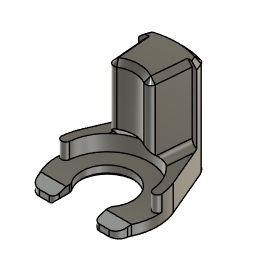
e3d_collet_clip (Autodesk Fusion 360 design; units mm, degrees)
Autodesk Fusion 360 part; units mm, degrees
sketch "Sketch1" plane through (0, 0, 0) normal (0, 0, 1) x (1, 0, 0)
  circle A0 centre (0, 0) radius 2.575
  circle A1 centre (0, 0) radius 5.0605
  line L0 (0, 0) -> (0, 7.5) construction
  line L1 (-2, -1.62192) -> (-2, -3.32192)
  line L2 (-4.4855, -2.342851) -> (-4.4855, -3.32192)
  line L3 (-4.4855, -3.32192) -> (-2, -3.32192)
  line L4 (4.4855, -2.342851) -> (4.4855, -3.32192)
  line L5 (4.4855, -3.32192) -> (2, -3.32192)
  line L6 (2, -1.62192) -> (2, -3.32192)
  arc A2 (2.5, 7.071068) -> (-2.5, 7.071068) centre (0, 0) ccw
  circle A3 centre (0, 0) radius 7.5 construction
  line L7 (-2.5, 7.071068) -> (-4.659517, 1.974223)
  line L8 (2.5, 7.071068) -> (4.659517, 1.974223)
  dimension "d1" = 5.15
  dimension "d2" = 2.4855
  dimension "d13" = 2.4855
  dimension "d18" = 2
  dimension "d20" = 1.7
  dimension "d37" = 15
  dimension "d41" = 5
  constraint coincident A0.centre A1.centre
  constraint concentric A0 A1
  constraint vertical L0
  constraint vertical L1
  constraint vertical L2
  constraint perpendicular L2 L3
  constraint concentric A2 A3
  constraint midpoint L0.end A2
  constraint tangent A1 L7
  constraint tangent A1 L8
  measures "d1" diameter of A0
  measures "d2" distance of A0 A1
  measures "d18" distance of L0 L1
  measures "d37" diameter of A3
extrude "Extrude1" add sketch "Sketch1" along normal blind 1 contours A0 A1 L1 L3 L5 L6 | A1 L2 L3 | A1 L4 L5 | A1 A2 L7 L8 picked at (2.605842, -2.755253) picked at (-4.279884, -3.007191) picked at (4.279884, -3.007191) picked at (0, 6.675289)
sketch "Sketch3" plane through (0, 0, 1) normal (0, 0, 1) x (-1, 0, 0)
  line L0 (2.5, -7.071068) -> (4.659517, -1.974223)
  arc A0 (4.659517, -1.974223) -> (4.4855, 2.342851) centre (0, 0) ccw
  line L1 (4.4855, 2.342851) -> (4.4855, 3.32192)
  line L2 (4.4855, 3.32192) -> (2, 3.32192)
  line L3 (2, 3.32192) -> (2, 1.62192)
  arc A1 (-2, 1.62192) -> (2, 1.62192) centre (0, 0) ccw
  line L4 (-2, 1.62192) -> (-2, 3.32192)
  line L5 (-2, 3.32192) -> (-4.4855, 3.32192)
  line L6 (-4.4855, 3.32192) -> (-4.4855, 2.342851)
  arc A2 (-4.4855, 2.342851) -> (-4.659517, -1.974223) centre (0, 0) ccw
  line L7 (-4.659517, -1.974223) -> (-2.5, -7.071068)
  arc A3 (-2.5, -7.071068) -> (2.5, -7.071068) centre (0, 0) ccw
  arc A4 (-2, 1.62192) -> (2, 1.62192) centre (0, 0) ccw
  arc A5 (-1.367588, -2.328025) -> (1.367588, -2.328025) centre (0, 0) ccw
  arc A6 (-4.185371, -0.3889) -> (4.185371, -0.3889) centre (0, 0) ccw
  arc A7 (5.038794, -0.4682) -> (4.185371, -0.3889) centre (4.612083, -0.42855) ccw
  arc A8 (-4.185371, -0.3889) -> (-5.038794, -0.4682) centre (-4.612083, -0.42855) ccw
  line L8 (5.0605, 0) -> (-5.0605, 0) construction
  line L9 (2.5, -7.071068) -> (2.118943, -2.715563)
  arc A9 (2.118943, -2.715563) -> (1.367588, -2.328025) centre (1.620845, -2.759141) ccw
  arc A10 (-1.367588, -2.328025) -> (-2.118943, -2.715563) centre (-1.620845, -2.759141) ccw
  line L10 (-2.118943, -2.715563) -> (-2.5, -7.071068)
  line L11 (2.5, -7.071068) -> (-2.5, -7.071068) construction
  line L12 (0, 0) -> (0, -7.071068) construction
  line L13 (-2, 1.62192) -> (-2, 3.32192)
  line L14 (2, 3.32192) -> (2, 1.62192)
  line L15 (2, 3.32192) -> (-2, 3.32192)
  line L16 (2.917598, -6.085463) -> (2.417598, -6.129207)
  line L17 (-2.417598, -6.129207) -> (-2.917598, -6.085463)
  dimension "d81" = 2.7
  dimension "d82" = 4.2034
  dimension "d108" = 85
  dimension "d109" = 0.5
  dimension "d125" = 0.5
  dimension "d127" = 0.42855
  constraint coincident A0.centre A1.centre
  constraint tangent A6 A7
  constraint tangent A0 A7
  constraint tangent A6 A8
  constraint tangent A2 A8
  constraint coincident A0 L8.start
  constraint coincident A2 L8.end
  constraint horizontal L8
  constraint coincident A0.centre L8
  constraint tangent A7 L8
  constraint tangent A8 L8
  constraint tangent L9 A9
  constraint tangent A5 A10
  constraint tangent A5 A9
  constraint tangent A10 L10
  constraint symmetric L9 L10 L12
  constraint symmetric A9 A10 L12
  constraint perpendicular L9 L16
  constraint perpendicular L10 L17
  constraint symmetric L12 L16 L17
  measures "d81" radius of A5
  measures "d82" radius of A6
  measures "d108" angle of L9 L11
  measures "d109" radius of A9
  measures "d127" radius of A7
extrude "Extrude5" add sketch "Sketch3" along normal blind 1.6 contours L0 L9 L16 | A3 A6 L9 L10 | L0 A0 A6 A7 L9 L16 | L7 L10 L17 | A2 L7 A6 A8 L10 L17 picked at (2.611732, -6.428579) picked at (-1.167502, -5.925234) picked at (3.545125, -3.647789) picked at (-2.611732, -6.428579) picked at (-3.545125, -3.647789)
extrude "Extrude6" add sketch "Sketch3" against normal up to surface (7.4 mm away) from surface at 9 contours L0 L9 L16 | A3 A6 L9 L10 | L7 L10 L17 | A5 A6 L9 A9 A10 L10 picked at (2.611732, -6.428579) picked at (-1.167502, -5.925234) picked at (-2.611732, -6.428579) picked at (-1.616583, -3.018571)
extrude "Extrude9" cut sketch "Sketch3" along normal blind 1.5 draft -45 from surface at 1.6 contours A0 L1 L2 L3 A1 L4 L5 L6 A2 A4 A5 A6 A7 A8 L9 A9 A10 L10 L13 L14 | A5 A6 L9 A9 A10 L10 | L3 A1 L4 A4 L13 L14 L15 picked at (2.8285, 2.428897) picked at (-1.616583, -3.018571) picked at (0.706619, -0.579754)
fillet "Fillet7" radius 0.5 4 edges at (2, -1.62192, 0.5) (2, -3.32192, 0.5) (-2, -3.32192, 0.5) (-2, -1.62192, 0.5)
fillet "Fillet8" radius 1 4 edges at (-4.4855, -3.32192, 0.5) (4.4855, -3.32192, 0.5) (-4.4855, -2.342851, 0.5) (4.4855, -2.342851, 0.5)
chamfer "Chamfer3" distance 1.2 distance2 0.4 2 edges at (3.000892, -3.32192, 1) (-3.000892, -3.32192, 1) measured on face at (-3.879636, -0.762521, 1) measured on face at (-3.879636, -0.762521, 1) tangent chain off
chamfer "Chamfer5" distance 0.3 angle 45 6 edges at (-2, -2.306173, 0) (-2.023947, -1.63754, 0) (0, 2.575, 0) (2.023947, -1.63754, 0) (2, -2.306173, 0) (0, 7.5, 0) tangent chain off
fillet "Fillet14" radius 0.7 2 edges at (-2.306293, 4.85699, 2.6) (2.306293, 4.85699, 2.6)
fillet "Fillet13" radius 0.5 2 edges at (2.5, 7.071068, 5.15) (-2.5, 7.071068, 5.15)
chamfer "Chamfer4" distance 0.5 angle 45 10 edges at (2.26827, 4.422385, 10) (1.850046, 2.314769, 10) (0, 2.7, 10) (-1.850046, 2.314769, 10) (-2.26827, 4.422385, 10) (-2.752673, 6.474716, 10) (-2.464293, 7.038339, 10) (0, 7.5, 10) (2.464293, 7.038339, 10) (2.752673, 6.474716, 10)
equation "d2 = e_width + 5 * e_spacing"
equation "d13 = d2"
equation "e_width = 0.45 mm"
equation "layer_height = 0.2 mm"
equation "e_spacing = 0.4071 mm"
equation "num_perimeters = 3"
equation "num_top_bottoms = 5"
equation "perimeters_width = e_width + ( num_perimeters - 1 ) * e_spacing"
equation "d127 = ( e_width + e_spacing ) / 2"
